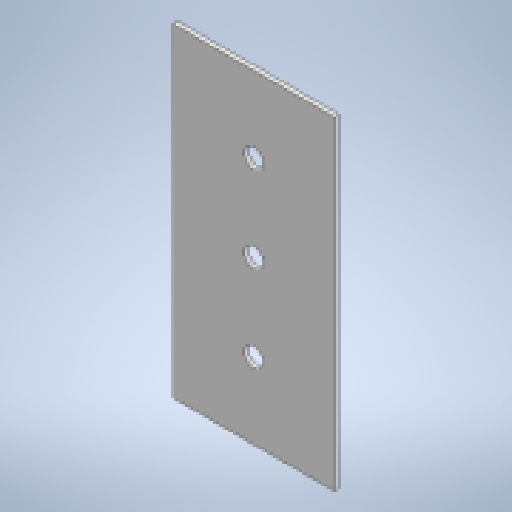
# Autodesk Inventor part: kosisita
Saved by Autodesk Inventor 2024 (Build 280153000, 153)
## iProperties
Created: 2024-07-10
Part Number: kosisita
Material: 一般
Document SubType Name: Modeling
Designer: right
Density: 1 g/cm^3
Appearance: 既定
Author: right
Autodesk Inventor part; units mm, degrees
ref_plane "YZ Plane" through (0, 0, 0) normal (1, 0, 0) x (0, 1, 0)
ref_plane "XZ Plane" through (0, 0, 0) normal (0, 1, 0) x (-1, 0, 0)
ref_plane "XY Plane" through (0, 0, 0) normal (0, 0, 1) x (1, 0, 0)
sketch "スケッチ1" plane through (0, 0, 0) normal (0, 0, 1) x (1, 0, 0)
  circle A0 centre (0, 0) radius 1.75 projected
  circle A1 centre (0, 0) radius 3
  circle A2 centre (0, -53.1322) radius 1.75 projected
  circle A3 centre (0, -53.1322) radius 3
  line L0 (0, 0) -> (0, -53.1322) construction
  circle A4 centre (0, -26.5661) radius 3
  line L1 (25, 23.4339) -> (-25, 23.4339)
  line L2 (-25, 23.4339) -> (-25, -76.5661)
  line L3 (-25, -76.5661) -> (25, -76.5661)
  line L4 (25, -76.5661) -> (25, 23.4339)
  line L5 (25, 23.4339) -> (-25, -76.5661) construction
  line L6 (-25, 23.4339) -> (25, -76.5661) construction
  point P0 (0, 0)
  dimension "d0" = 6
  dimension "d1" = 6
  dimension "d2" = 6
  dimension "d3" = 100
  dimension "d4" = 50
  constraints: 14 end point, 3 centre point, 3 midpoint, 2 coincident, 2 parallel, 1 horizontal, 1 perpendicular, 1 vertical
  measures "d0" diameter of A1
  measures "d1" diameter of A3
  measures "d2" diameter of A4
  measures "d3" distance of L3.end L1.start
  measures "d4" distance between parallel lines of L2 L4
extrude "押し出し1" add sketch "スケッチ1" along normal blind 1.5 contours L4 L3 L2 L1
